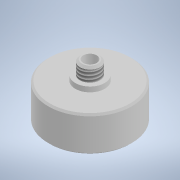
# Autodesk Inventor part: 191203 ESF-4A
Saved by Autodesk Inventor 2021 (Build 250183000, 183)
## iProperties
Created: 2026-04-25
Part Number: 191203 ESF-4A
Material: Generic
Catalog Web Link: www.3dfindit.com
Description: ESF-vacuum filter
Vendor: FESTO
Document SubType Name: Modeling
Designer: psAdmin
Manufacturer: FESTO
Mass: 19 g
Surface Area: 20.2664 cm^2
Volume: 5.15035 cm^3
Density: 1 g/cm^3
Appearance: PSOLRGB-176-176-176
Category: PARTsolutions
Company: FESTO
Title: 191203 ESF-4A
Author: Cadenas PARTsolutions
Comments: vacuum filter
PSOL_IDENT_0: {$CADENAS_DATA/23d-libs/festo/parts/e/esf/esf.prj},163 {VTYP=3D},{NB=191203 ESF-4A},{LINA=191203 ESF
PSOL_IDENT_1: -4A},{NN=ESF},{DATE=02.05.2025 09:04:04},{GEOMDATE=19.03.2025 08:29:22},{VERSION=},{LINEID=20},{WBVA
PSOL_IDENT_2: R=},{WBNUMERIC=}  {NB=191203 ESF-4A},{LINA=191203 ESF-4A},{KT=0},{TNR=191203},{TYP=ESF-4A},{D1=25.00
PSOL_IDENT_3: 0},{D2=M6},{D2N=6.000},{D3=8.800},{L1=10.500},{L2=5.500},{L3=4.000},{GR=0.000},{ZZ=0.001},{NENN=4A},
PSOL_IDENT_4: {GRN=20.000},{CNSMASSEXACT=0.019},{GTIN=4052568079192},{REACH=Ja},{REACHSVHC=Ja},{REACHHAZSUBS=7439-
PSOL_IDENT_5: 92-1},{REACHSCIP=17c6562e-c284-49a6-a1b0-4e46ba5d1ac8},{REACHVALDATE=05.03.2025}
NB: 191203 ESF-4A
NN: ESF
NT: vacuum filter
NBSYN: $TNR. $TYP.
LINA: 191203 ESF-4A
CATALOG: Festo
TNR: 191203
TYP: ESF-4A
D1: 25
D2: M6
D3: 8.8
L1: 10.5
L2: 5.5
L3: 4
CNSMASSEXACT: 0.019
GTIN: 4052568079192
REACH: Yes
REACHSVHC: Yes
REACHHAZSUBS: 7439-92-1
REACHVALDATE: 05.03.2025
SUPPLIER: FESTO
ARTICLENO: 191203 ESF-4A
BOMINFO: 191203 ESF-4A
CREATOR: CADENAS GmbH
Autodesk Inventor part; units mm, degrees
sketch "Sketch_6" plane through (0, 0, 0) normal (0, 0, 1) x (1, 0, 0)
  line L0 (0, 0) -> (0, 16)
  line L1 (0, 16) -> (2.3865, 16)
  line L2 (2.3865, 16) -> (3, 15.3865)
  line L3 (3, 15.3865) -> (3, 12)
  line L4 (3, 12) -> (4.4, 12)
  line L5 (4.4, 12) -> (4.4, 10.5)
  line L6 (4.4, 10.5) -> (12, 10.5)
  line L7 (12, 10.5) -> (12.5, 10)
  line L8 (12.5, 10) -> (12.5, 0.5)
  line L9 (12.5, 0.5) -> (12, 0)
  line L10 (12, 0) -> (0, 0)
  line L11 (0, 0) -> (0, 16)
  constraints: 24 end point
revolve "Revolution1" add sketch "Sketch_6" angle 360 about axis through (0, 0, 0) along (0, 1, 0)
thread "Thread1" size "M6x1" class "6g" standard "ISO Metric profile" full length
sketch "Sketch_4" plane through (0, 0, 0) normal (0, 0, 1) x (1, 0, 0)
  line L0 (0, 0) -> (0, 6)
  line L1 (0, 6) -> (2.4585, 6)
  line L2 (2.4585, 6) -> (2.4585, 0.5415)
  line L3 (2.4585, 0.5415) -> (3, 0)
  line L4 (3, 0) -> (0, 0)
  line L5 (0, 0) -> (0, 6)
  constraints: 12 end point
revolve "Revolution2" cut sketch "Sketch_4" angle 360 about axis through (0, 0, 0) along (0, -1, 0)
thread "Thread2" size "M6x1" class "6H" standard "ISO Metric profile" full length
sketch "Sketch_5" plane through (0, 0, 0) normal (0, 0, 1) x (1, 0, 0)
  line L0 (0, 10.5) -> (0, 16)
  line L1 (0, 16) -> (2, 16)
  line L2 (2, 16) -> (2, 10.5)
  line L3 (2, 10.5) -> (0, 10.5)
  line L4 (0, 10.5) -> (0, 16)
  constraints: 10 end point
revolve "Revolution3" cut sketch "Sketch_5" angle 360 about axis through (0, 10.5, 0) along (0, -1, 0)
ref_plane "oben_XY" through (0, 12, 0) normal (0, 1, 0) x (1, 0, 0)
ref_plane "oben_YZ" through (0, 12, 0) normal (1, 0, 0) x (0, 0, -1)
ref_plane "oben_ZX" through (0, 12, 0) normal (0, 0, -1) x (0, 1, 0)
ref_plane "unten_XY" through (0, 0, 0) normal (0, 1, 0) x (1, 0, 0)
ref_plane "unten_YZ" through (0, 0, 0) normal (1, 0, 0) x (0, 0, -1)
ref_plane "unten_ZX" through (0, 0, 0) normal (0, 0, -1) x (0, 1, 0)
body "Solid1"
